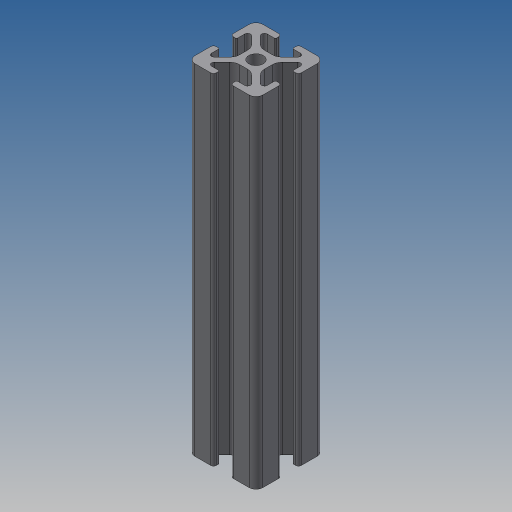
# Autodesk Inventor part: Item_0037003-100
Saved by Autodesk Inventor 2024.3 (Build 283343000, 343)
## iProperties
Created: 2020-04-29
Part Number: Item_0037003-100
Project: Source
Material: .
Description: Profil 5 20x20x100
Document SubType Name: Modeling
Designer: JVY
Authority: 20x20xL
Density: 0.001 g/cm^3
Appearance: Par défaut
Mass: 0.0183852 g
Surface Area: 172.792 cm^2
Volume: 18.3852 cm^3
Material number: ---
Author: JVY
Autodesk Inventor part; units mm, degrees
ref_plane "Plan YZ" through (0, 0, 0) normal (1, 0, 0) x (0, 1, 0)
ref_plane "Plan XZ" through (0, 0, 0) normal (0, 1, 0) x (-1, 0, 0)
ref_plane "Plan XY" through (0, 0, 0) normal (0, 0, 1) x (1, 0, 0)
sketch "Esquisse1" plane through (0, 0, 0) normal (0, 0, 1) x (1, 0, 0)
  line L0 (6.779, -5.5062) -> (4.5287, -3.2559)
  line L1 (-4.5287, 3.2559) -> (-6.779, 5.5062)
  line L2 (5.5062, -6.779) -> (3.2559, -4.5287)
  line L3 (-3.2559, 4.5287) -> (-5.5062, 6.779)
  line L4 (3.3, -10) -> (8, -10)
  line L5 (-8, -10) -> (-3.3, -10)
  line L6 (-4.9176, -8.2) -> (-2.8, -8.2)
  line L7 (2.8, -8.2) -> (4.9176, -8.2)
  line L8 (-1.1346, -3.65) -> (1.1346, -3.65)
  line L9 (8.5, -2.5) -> (9.2, -2.5)
  line L10 (-9.2, -2.5) -> (-8.5, -2.5)
  line L11 (8.5, 2.5) -> (9.2, 2.5)
  line L12 (-9.2, 2.5) -> (-8.5, 2.5)
  line L13 (-1.1346, 3.65) -> (1.1346, 3.65)
  line L14 (2.8, 8.2) -> (4.9176, 8.2)
  line L15 (-4.9176, 8.2) -> (-2.8, 8.2)
  line L16 (3.3, 10) -> (8, 10)
  line L17 (-8, 10) -> (-3.3, 10)
  line L18 (4.5287, 3.2559) -> (6.779, 5.5062)
  line L19 (-5.5062, -6.779) -> (-3.2559, -4.5287)
  line L20 (3.2559, 4.5287) -> (5.5062, 6.779)
  line L21 (-6.779, -5.5062) -> (-4.5287, -3.2559)
  line L22 (-10, 3.3) -> (-10, 8)
  line L23 (-10, -8) -> (-10, -3.3)
  line L24 (-8.2, 2.8) -> (-8.2, 4.9176)
  line L25 (-8.2, -4.9176) -> (-8.2, -2.8)
  line L26 (-3.65, -1.1346) -> (-3.65, 1.1346)
  line L27 (-2.5, 8.5) -> (-2.5, 9.2)
  line L28 (-2.5, -9.2) -> (-2.5, -8.5)
  line L29 (2.5, -9.2) -> (2.5, -8.5)
  line L30 (2.5, 8.5) -> (2.5, 9.2)
  line L31 (3.65, -1.1346) -> (3.65, 1.1346)
  line L32 (8.2, -4.9176) -> (8.2, -2.8)
  line L33 (8.2, 2.8) -> (8.2, 4.9176)
  line L34 (10, -8) -> (10, -3.3)
  line L35 (10, 3.3) -> (10, 8)
  arc A0 (-9.2, -2.5) -> (-10, -3.3) centre (-9.2, -3.3) ccw
  arc A1 (-10, 3.3) -> (-9.2, 2.5) centre (-9.2, 3.3) ccw
  arc A2 (-8.2, -2.8) -> (-8.5, -2.5) centre (-8.5, -2.8) ccw
  arc A3 (-8.5, 2.5) -> (-8.2, 2.8) centre (-8.5, 2.8) ccw
  arc A4 (-10, -8) -> (-8, -10) centre (-8, -8) ccw
  arc A5 (-8, 10) -> (-10, 8) centre (-8, 8) ccw
  arc A6 (-8.2, -4.9176) -> (-6.779, -5.5062) centre (-7.3676, -4.9176) ccw
  arc A7 (-6.779, 5.5062) -> (-8.2, 4.9176) centre (-7.3676, 4.9176) ccw
  arc A8 (-4.5287, -3.2559) -> (-3.65, -1.1346) centre (-6.65, -1.1346) ccw
  arc A9 (-3.65, 1.1346) -> (-4.5287, 3.2559) centre (-6.65, 1.1346) ccw
  arc A10 (-5.5062, -6.779) -> (-4.9176, -8.2) centre (-4.9176, -7.3676) ccw
  arc A11 (-4.9176, 8.2) -> (-5.5062, 6.779) centre (-4.9176, 7.3676) ccw
  arc A12 (-3.3, -10) -> (-2.5, -9.2) centre (-3.3, -9.2) ccw
  arc A13 (-2.5, 9.2) -> (-3.3, 10) centre (-3.3, 9.2) ccw
  arc A14 (-2.5, -8.5) -> (-2.8, -8.2) centre (-2.8, -8.5) ccw
  arc A15 (-2.8, 8.2) -> (-2.5, 8.5) centre (-2.8, 8.5) ccw
  arc A16 (-1.1346, -3.65) -> (-3.2559, -4.5287) centre (-1.1346, -6.65) ccw
  arc A17 (-3.2559, 4.5287) -> (-1.1346, 3.65) centre (-1.1346, 6.65) ccw
  circle A18 centre (0, 0) radius 2.15
  arc A19 (3.2559, -4.5287) -> (1.1346, -3.65) centre (1.1346, -6.65) ccw
  arc A20 (1.1346, 3.65) -> (3.2559, 4.5287) centre (1.1346, 6.65) ccw
  arc A21 (2.8, -8.2) -> (2.5, -8.5) centre (2.8, -8.5) ccw
  arc A22 (2.5, 8.5) -> (2.8, 8.2) centre (2.8, 8.5) ccw
  arc A23 (2.5, -9.2) -> (3.3, -10) centre (3.3, -9.2) ccw
  arc A24 (3.3, 10) -> (2.5, 9.2) centre (3.3, 9.2) ccw
  arc A25 (4.9176, -8.2) -> (5.5062, -6.779) centre (4.9176, -7.3676) ccw
  arc A26 (5.5062, 6.779) -> (4.9176, 8.2) centre (4.9176, 7.3676) ccw
  arc A27 (3.65, -1.1346) -> (4.5287, -3.2559) centre (6.65, -1.1346) ccw
  arc A28 (4.5287, 3.2559) -> (3.65, 1.1346) centre (6.65, 1.1346) ccw
  arc A29 (6.779, -5.5062) -> (8.2, -4.9176) centre (7.3676, -4.9176) ccw
  arc A30 (8.2, 4.9176) -> (6.779, 5.5062) centre (7.3676, 4.9176) ccw
  arc A31 (8, -10) -> (10, -8) centre (8, -8) ccw
  arc A32 (10, 8) -> (8, 10) centre (8, 8) ccw
  arc A33 (8.5, -2.5) -> (8.2, -2.8) centre (8.5, -2.8) ccw
  arc A34 (8.2, 2.8) -> (8.5, 2.5) centre (8.5, 2.8) ccw
  arc A35 (10, -3.3) -> (9.2, -2.5) centre (9.2, -3.3) ccw
  arc A36 (9.2, 2.5) -> (10, 3.3) centre (9.2, 3.3) ccw
  constraints: 72 end point, 72 point on circle, 37 centre point, 14 horizontal, 14 vertical, 155 other
extrude "Extrusion1" add sketch "Esquisse1" along normal blind 100
